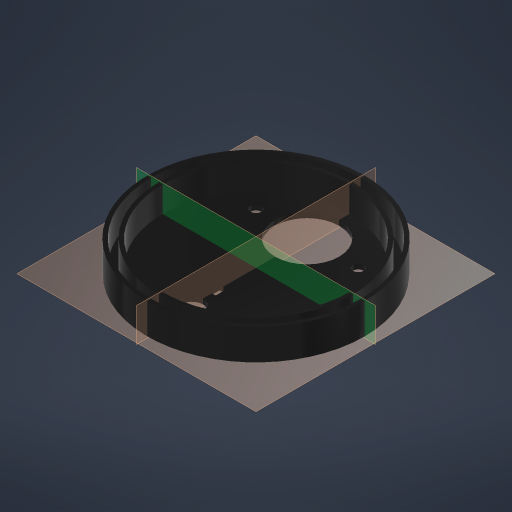
# Autodesk Inventor part: Reservoir Adapter
Saved by Autodesk Inventor 2024 (Build 280153000, 153)
## iProperties
Manager: Louis Van Roosmaelen
Company: DCS - DIGITAL COMBAT SIMULATOR
Created: 2023-11-02
Part Number: Reservoir Adapter
Material: S235
Catalog Web Link: http://emmausbovenbouw.op-weg.be/
Vendor: Emmaüsinstituut Bovenbouw Aalter
Document SubType Name: Modeling
Designer: Louis
Engineer: Declercq St.
Manufacturer: Standard
Standards Organization: Custom
Density: 7.86 g/cm^3
Appearance: Smooth - Black
IDENT.NR.: AJ2022
TEAM: 30
Title: F18C Home Cockpit
Author: Louis
Keywords: Ø
Autodesk Inventor part; units mm, degrees
sketch "Sketch1" plane through (0, 0, 0) normal (0, 0, 1) x (1, 0, 0)
  line L0 (0, 2.8582) -> (0, -2.8582) construction
  line L1 (-5.7775, 0) -> (5.7775, 0) construction
  circle A0 centre (0, 0) radius 42.5
  dimension "d0" = 85
  constraints: 4 end point, 2 coincident, 2 midpoint, 1 centre point, 1 horizontal, 1 vertical
  measures "d0" diameter of A0
extrude "Extrusion1" add sketch "Sketch1" along normal blind 2
sketch "Sketch2" plane through (0, 0, 2) normal (0, 0, 1) x (1, 0, 0)
  circle A0 centre (0, 0) radius 41
  circle A1 centre (0, 0) radius 38
  circle A2 centre (0, 0) radius 42.5 projected
  circle A3 centre (0, 0) radius 36.5
  dimension "d3" = 82
  dimension "d4" = 76
  dimension "d5" = 73
  constraints: 3 centre point, 3 coincident
  measures "d3" diameter of A0
  measures "d4" diameter of A1
  measures "d5" diameter of A3
extrude "Extrusion2" add sketch "Sketch2" along normal blind 10
sketch "Sketch3" plane through (0, 0, 0) normal (0, 0, -1) x (-1, 0, 0)
  circle A0 centre (0, 0) radius 42.5 projected
  circle A1 centre (0, -25) radius 4.25
  line L0 (-59.5, 0) -> (59.5, 0) projected
  line L1 (1.5, -17.25) -> (-1.5, -17.25)
  line L2 (-1.5, -17.25) -> (-1.5, -12.75)
  line L3 (-1.5, -12.75) -> (1.5, -12.75)
  line L4 (1.5, -12.75) -> (1.5, -17.25)
  line L5 (1.5, -17.25) -> (-1.5, -12.75) construction
  line L6 (-1.5, -17.25) -> (1.5, -12.75) construction
  line L7 (0, -59.5) -> (0, 59.5) projected
  circle A2 centre (0, 20) radius 12.5
  point P0 (0, -15)
  dimension "d8" = 8.5
  dimension "d9" = 25
  dimension "d11" = 3
  dimension "d12" = 4.5
  dimension "d13" = 15
  dimension "d14" = 25
  dimension "d15" = 20
  constraints: 12 end point, 3 point on line, 2 centre point, 2 midpoint, 2 parallel, 1 horizontal, 1 perpendicular
  measures "d8" diameter of A1
  measures "d9" distance from line of L0 A1.centre
  measures "d11" distance of L2.end L3.end
  measures "d12" distance of L1.end L2.end
  measures "d13" distance of point (0, 0) point (0, -15)
  measures "d14" diameter of A2
  measures "d15" distance from line of L0 A2.centre
extrude "Extrusion3" cut sketch "Sketch3" against normal up to surface (2 mm away) contours A2 L7 | L7 A2 | L7 A1 | A1 L7 | L7 L1 L2 L3 | L3 L4 L1 L7
sketch "Sketch4" plane through (0, 0, 0) normal (0, 0, -1) x (-1, 0, 0)
  circle A0 centre (0, -25) radius 4.25 projected
  circle A1 centre (0, 20) radius 12.5 projected
  line L0 (1.5, -12.75) -> (-1.5, -12.75) projected
  line L1 (-1.5, -12.75) -> (-1.5, -17.25) projected
  line L2 (-1.5, -17.25) -> (1.5, -17.25) projected
  line L3 (1.5, -17.25) -> (1.5, -12.75) projected
  circle A2 centre (0, 0) radius 42.5 projected
  line L4 (-59.5, 0) -> (59.5, 0) projected
  point P0 (-20, 20)
  point P1 (20, 20)
  dimension "d18" = 20
  dimension "d19" = 20
  dimension "d20" = 20
  dimension "d21" = 20
  measures "d18" distance of A1.centre point (20, 20)
  measures "d19" distance of point (-20, 20) A1.centre
  measures "d20" distance from line of L4 point (-20, 20)
  measures "d21" distance from line of L4 point (20, 20)
hole "Hole1" at (20, 20, 0) at (-20, 20, 0) direction (0, 0, 1) diameter 4.2 end through all
body "Solid1"
